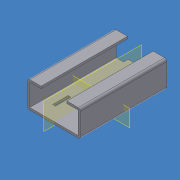
# Autodesk Inventor part: 90-05-089
Saved by Autodesk Inventor 2015 SP1 (Build 190203100, 203)
## iProperties
Created: 2007-07-03
Part Number: 90-05-089
Material: Steel, Mild
Document SubType Name: Sheet Metal
Designer: kurt
Manufacturer: Standard
Standards Organization: Custom
Density: 1 g/cm^3
Sheet Metal Rule: Default
Appearance: Steel
Author: kurt
Autodesk Inventor part; units mm, degrees
ref_plane "YZ Plane" through (0, 0, 0) normal (1, 0, 0) x (0, 1, 0)
ref_plane "XZ Plane" through (0, 0, 0) normal (0, 1, 0) x (-1, 0, 0)
ref_plane "XY Plane" through (0, 0, 0) normal (0, 0, 1) x (1, 0, 0)
sketch "Sketch1" plane through (0, 0, 0) normal (0, 0, 1) x (1, 0, 0)
  line L0 (-32, 0) -> (32, 0)
  line L1 (32, 0) -> (32, 114)
  line L2 (-32, 114) -> (-32, 0)
  line L3 (-22, 114) -> (-22, 120)
  line L4 (-22, 120) -> (22, 120)
  line L5 (22, 120) -> (22, 114)
  line L6 (32, 114) -> (22, 114)
  line L7 (-22, 114) -> (-32, 114)
  point P0 (0, 0)
  point P1 (0, 0)
  dimension "d42" = 114
  dimension "d49" = 10
  dimension "d50" = 10
  dimension "d51" = 6
  dimension "d52" = 64
  dimension "d53" = 64
  measures "d42" distance of L0.end L1.end
  measures "d49" horizontal distance of L2.start L3.end
  measures "d50" horizontal distance of L1.end L4.end
  measures "d51" distance of L3.start L3.end
  measures "d52" distance of L1.end L2.start
  measures "d53" distance of L0.end L0.start
extrude "Plate1" add sketch "Sketch1" along normal blind 3
sketch "Sketch2" plane through (-32, 0, 3) normal (1, 0, 0) x (0, 1, 0)
  line L0 (0, 0) -> (114, 0)
  line L1 (114, 0) -> (114, 29)
  line L2 (114, 29) -> (0, 29)
  line L3 (0, 29) -> (0, 0)
  constraints: 6 end point, 1 horizontal, 1 perpendicular, 1 vertical
sheet face with bend "Flange1" sketch "Sketch2" thickness 3 toward (-1, 0, 0) bend radius 0.001 relief straight relief width 3 relief depth 0.001
bend "Bend1"
sketch "Sketch3" plane through (32, 114, 3) normal (-1, 0, 0) x (0, -1, 0)
  line L0 (0, 0) -> (114, 0)
  line L1 (114, 0) -> (114, 29)
  line L2 (114, 29) -> (0, 29)
  line L3 (0, 29) -> (0, 0)
  constraints: 6 end point, 1 horizontal, 1 perpendicular, 1 vertical
sheet face with bend "Flange2" sketch "Sketch3" thickness 3 toward (1, 0, 0) bend radius 0.001 relief straight relief width 3 relief depth 0.001
bend "Bend2"
sketch "Sketch4" plane through (-32, 0, 32) normal (0, 0, -1) x (0, 1, 0)
  line L0 (0, 0) -> (114, 0)
  line L1 (114, 0) -> (114, 15)
  line L2 (114, 15) -> (0, 15)
  line L3 (0, 15) -> (0, 0)
  constraints: 6 end point, 1 horizontal, 1 perpendicular, 1 vertical
sheet face with bend "Flange3" sketch "Sketch4" thickness 3 toward (0, 0, 1) bend radius 0.001 relief straight relief width 3 relief depth 0.001
bend "Bend3"
sketch "Sketch5" plane through (32, 114, 32) normal (0, 0, -1) x (0, -1, 0)
  line L0 (0, 0) -> (114, 0)
  line L1 (114, 0) -> (114, 15)
  line L2 (114, 15) -> (0, 15)
  line L3 (0, 15) -> (0, 0)
  constraints: 6 end point, 1 horizontal, 1 perpendicular, 1 vertical
sheet face with bend "Flange4" sketch "Sketch5" thickness 3 toward (0, 0, 1) bend radius 0.001 relief straight relief width 3 relief depth 0.001
bend "Bend4"
ref_plane "Work Plane7" through (31.999, 57, 0) normal (0, 1, 0) x (-1, 0, 0)
sketch "Sketch6" plane through (-31.999, 0, 0) normal (0, 0, -1) x (-1, 0, 0)
  line L0 (-11.499, 39) -> (-15.499, 39)
  line L1 (-15.499, 39) -> (-15.499, 18.5)
  line L2 (-15.499, 18.5) -> (-11.499, 18.5)
  line L3 (-11.499, 18.5) -> (-11.499, 39)
  line L4 (-31.999, -12) -> (-31.999, 156) construction
  line L5 (-48.499, 18.5) -> (-52.499, 18.5)
  line L6 (-52.499, 18.5) -> (-52.499, 39)
  line L7 (-52.499, 39) -> (-48.499, 39)
  line L8 (-48.499, 39) -> (-48.499, 18.5)
  circle A0 centre (-31.999, 35) radius 4.5
  line L9 (-87.999, 57) -> (10.001, 57) projected
  line L10 (0, 0) -> (-63.998, 0) projected
  dimension "d33" = 4
  dimension "d34" = 20.5
  dimension "d35" = 4
  dimension "d36" = 20.5
  dimension "d37" = 0
  dimension "d38" = 33
  dimension "d46" = 9
  dimension "d47" = 0
  dimension "d48" = 4
  dimension "d56" = 18.5
  constraints: 16 end point, 4 parallel, 2 horizontal, 2 perpendicular, 1 centre point, 1 other
  measures "d33" distance of L0.start L0.end
  measures "d34" distance of L2.end L0.start
  measures "d35" distance of L6.end L7.end
  measures "d36" distance of L5.end L6.end
  measures "d37" vertical distance of L0.end L7.end
  measures "d38" distance of L5.start L1.end
  measures "d46" diameter of A0
  measures "d47" distance from line of L4 A0.centre
  measures "d48" vertical distance of L0.end A0.centre
  measures "d56" distance from line of L10 L2.end
extrude "Cut1" cut sketch "Sketch6" against normal blind 4
ref_plane "Work Plane6" through (0, 0, 3) normal (1, 0, 0) x (0, 0, -1)
equation "\"d5\" = BendReliefWidth"
equation "\"d7\" = MinimumRemnant"
equation "\"d11\" = BendRadius"
equation "\"d6\" = BendReliefDepth"
equation "\"d8\" = BendRadius"
equation "\"d12\" = BendReliefWidth"
equation "\"d14\" = MinimumRemnant"
equation "\"d18\" = BendRadius"
equation "\"d13\" = BendReliefDepth"
equation "\"d15\" = BendRadius"
equation "\"d19\" = BendReliefWidth"
equation "\"d21\" = MinimumRemnant"
equation "\"d25\" = BendRadius"
equation "\"d20\" = BendReliefDepth"
equation "\"d22\" = BendRadius"
equation "\"d26\" = BendReliefWidth"
equation "\"d28\" = MinimumRemnant"
equation "\"d32\" = BendRadius"
equation "\"d27\" = BendReliefDepth"
equation "\"d29\" = BendRadius"
equation "\"BendReliefWidth\" = Thickness"
equation "\"CornerReliefSize\" = 4 * Thickness"
equation "\"MinimumRemnant\" = 2 * Thickness"
equation "\"TransitionRadius\" = BendRadius"
equation "\"d4\" = BendRadius"
equation "\"JacobiRadiusSize\" = Thickness"
equation "\"GapSize\" = Thickness"
equation "\"BendRadius\" = 0.001"
equation "\"BendReliefDepth\" = 0.001"
equation "\"Thickness\" = 3"
body "Solid1"
